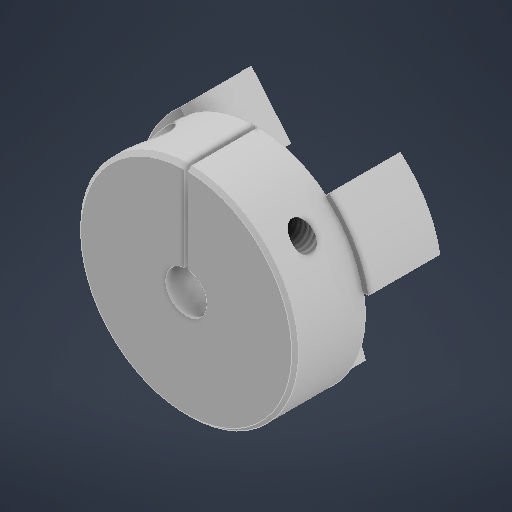
# Autodesk Inventor part: Coupling
Saved by Autodesk Inventor 2027 (Build 310192000, 192)
## iProperties
Category: PARTsolutions
Company: FESTO
Created: 2026-05-27
Part Number: Coupling
Material: Generic
Catalog Web Link: www.3dfindit.com
Description: EAMD-coupling
Vendor: FESTO
Document SubType Name: Modeling
Designer: psAdmin
Manufacturer: FESTO
Mass: 126 g
Surface Area: 117.587 cm^2
Volume: 24.6259 cm^3
Density: 1 g/cm^3
Appearance: PSOLRGB-176-176-176
PSOL_IDENT_0: {$CADENAS_DATA/23d-libs/festo/parts/e/eamd/eamd.prj},190 {VTYP=3D},{NB=558001 EAMD-32-32-11-16x20},{
PSOL_IDENT_1: LINA=558001 EAMD-32-32-11-16x20},{NN=EAMD},{DATE=05.05.2026 07:51:46},{GEOMDATE=01.09.2025 08:29:23}
PSOL_IDENT_2: ,{VERSION=},{LINEID=40},{WBVAR=},{WBNUMERIC=}  {NB=558001 EAMD-32-32-11-16x20},{LINA=558001 EAMD-32-
PSOL_IDENT_3: 32-11-16x20},{KT=DUMMY},{TNR=558001},{TYP=EAMD-32-32-11-16x20},{INFO=},{D1=11.000},{D2=16.000},{DA=0
PSOL_IDENT_4: .000},{F=0.000},{L1=0.000},{L2=0.000},{L3=0.000},{L4=0.000},{L5=0.000},{A=3.950},{VERS=3},{CNSMASSEX
PSOL_IDENT_5: ACT=0.1260},{GTIN=4052568204419},{EOLDATE=}
NB: 558001 EAMD-32-32-11-16x20
NN: EAMD
NT: coupling
NBSYN: $TNR. $TYP.
LINA: 558001 EAMD-32-32-11-16x20
CATALOG: Festo
TNR: 558001
TYP: EAMD-32-32-11-16x20
D1: 11
D2: 16
DA: 0
F: 0
L1: 0
L2: 0
L3: 0
L4: 0
L5: 0
CNSMASSEXACT: 0.126
GTIN: 4052568204419
SUPPLIER: FESTO
ARTICLENO: 558001 EAMD-32-32-11-16x20
BOMINFO: 558001 EAMD-32-32-11-16x20
CREATOR: CADENAS GmbH
Title: 558001 EAMD-32-32-11-16x20
Author: Cadenas PARTsolutions
Comments: coupling
Autodesk Inventor part; units mm, degrees
sketch "Sketch_1" plane through (0, 0, 0) normal (1, 0, 0) x (0, 1, 0)
  line L0 (0, -10.3) -> (0, 0)
  line L1 (0, 0) -> (15.5, 0)
  line L2 (15.5, 0) -> (16, -0.5)
  line L3 (16, -0.5) -> (16, -10.3)
  line L4 (16, -10.3) -> (0, -10.3)
  line L5 (0, -10.3) -> (0, 0)
  constraints: 12 end point
revolve "Revolution1" add sketch "Sketch_1" angle 360 about axis through (0, 0, -10.3) along (0, 0, -1)
sketch "Sketch_2" plane through (0, 0, -10.1) normal (0, 0, 1) x (1, 0, 0)
  line L0 (-16.7417, 2.952) -> (-7.8785, 1.3892)
  arc A0 (-5.1423, 6.1284) -> (-7.8785, 1.3892) centre (0, 0) ccw
  line L1 (-5.1423, 6.1284) -> (-10.9274, 13.0228)
  arc A1 (-10.9274, 13.0228) -> (-16.7417, 2.952) centre (0, 0) ccw
  constraints: 4 end point, 4 point on circle, 2 centre point
extrude "Extrusion1" add sketch "Sketch_2" against normal blind 10.4
sketch "Sketch_3" plane through (0, 0, -10.1) normal (0, 0, 1) x (1, 0, 0)
  arc A0 (-5.8143, -15.9748) -> (5.8143, -15.9748) centre (0, 0) ccw
  line L0 (5.8143, -15.9748) -> (2.7362, -7.5175)
  arc A1 (-2.7362, -7.5175) -> (2.7362, -7.5175) centre (0, 0) ccw
  line L1 (-2.7362, -7.5175) -> (-5.8143, -15.9748)
  constraints: 4 end point, 4 point on circle, 2 centre point
extrude "Extrusion2" add sketch "Sketch_3" against normal blind 10.4
sketch "Sketch_19" plane through (0, 0, -10.1) normal (0, 0, 1) x (1, 0, 0)
  arc A0 (7.8785, 1.3892) -> (5.1423, 6.1284) centre (0, 0) ccw
  line L0 (7.8785, 1.3892) -> (16.7417, 2.952)
  arc A1 (16.7417, 2.952) -> (10.9274, 13.0228) centre (0, 0) ccw
  line L1 (10.9274, 13.0228) -> (5.1423, 6.1284)
  constraints: 4 end point, 4 point on circle, 2 centre point
extrude "Extrusion3" add sketch "Sketch_19" against normal blind 10.4
sketch "Sketch_9" plane through (0, 0, 0) normal (1, 0, 0) x (0, 1, 0)
  line L0 (0, -28.3636) -> (0, 0)
  line L1 (0, 0) -> (3, 0)
  line L2 (3, 0) -> (3, -5.5091)
  line L3 (3, -5.5091) -> (3.8727, -5.5091)
  line L4 (3.8727, -5.5091) -> (3.8727, -11.8909)
  line L5 (3.8727, -11.8909) -> (2.4545, -11.8909)
  line L6 (2.4545, -11.8909) -> (2.4545, -13.2545)
  line L7 (2.4545, -13.2545) -> (1.1275, -13.2545)
  line L8 (1.1275, -13.2545) -> (1.1275, -28.1275)
  line L9 (1.1275, -28.1275) -> (1.3636, -28.3636)
  line L10 (1.3636, -28.3636) -> (0, -28.3636)
  line L11 (0, -28.3636) -> (0, 0)
  dimension "d36" = 3
  constraints: 24 end point
  measures "d36" distance of L1.start L1.end
revolve "Revolution3" cut sketch "Sketch_9" angle 360 about axis through (0, 0, -28.3636) along (0, 0, -1)
sketch "Sketch_12" plane through (0, 0, 0) normal (0, 0, 1) x (1, 0, 0)
  line L0 (-0.25, 16) -> (-0.25, 0)
  line L1 (-0.25, 0) -> (0.25, 0)
  line L2 (0.25, 0) -> (0.25, 16)
  line L3 (0.25, 16) -> (-0.25, 16)
  constraints: 8 end point
extrude "Extrusion10" cut sketch "Sketch_12" against normal blind 10.1
sketch "Sketch_13" plane through (0, 0, -5.1) normal (0, 0, 1) x (1, 0, 0)
  line L0 (13.5, 10.5) -> (-16.5, 10.5)
  line L1 (-16.5, 10.5) -> (-16.5, 14.1)
  line L2 (-16.5, 14.1) -> (-4.5, 14.1)
  line L3 (-4.5, 14.1) -> (-4.5, 12.5)
  line L4 (-4.5, 12.5) -> (-4.121, 12.121)
  line L5 (-4.121, 12.121) -> (13.5, 12.121)
  line L6 (13.5, 12.121) -> (13.5, 10.5)
  line L7 (13.5, 10.5) -> (-16.5, 10.5)
  constraints: 16 end point
revolve "Revolution6" cut sketch "Sketch_13" angle 360 about axis through (13.5, 10.5, -5.1) along (-1, 0, 0)
thread "Thread2" size "M4x0.7" class "6H" standard "ISO Metric profile" length 17.621
sketch "Sketch_11" plane through (0, 0, -21.8) normal (0, 0, 1) x (0, 1, 0)
  arc A0 (-1.8674, -0.5726) -> (-1.4296, -1.3309) centre (-1.5586, -0.8998) ccw
  arc A1 (-0.4378, -1.9035) -> (-1.4296, -1.3309) centre (-1.2039, -2.0852) ccw
  arc A2 (-0.4378, -1.9035) -> (0.4378, -1.9035) centre (0, -1.7997) ccw
  arc A3 (1.4296, -1.3309) -> (0.4378, -1.9035) centre (1.2039, -2.0852) ccw
  arc A4 (1.4296, -1.3309) -> (1.8674, -0.5726) centre (1.5586, -0.8998) ccw
  arc A5 (1.8674, 0.5726) -> (1.8674, -0.5726) centre (2.4078, 0) ccw
  arc A6 (1.8674, 0.5726) -> (1.4296, 1.3309) centre (1.5586, 0.8999) ccw
  arc A7 (0.4378, 1.9035) -> (1.4296, 1.3309) centre (1.2039, 2.0852) ccw
  arc A8 (0.4378, 1.9035) -> (-0.4378, 1.9035) centre (0, 1.7997) ccw
  arc A9 (-1.4296, 1.3309) -> (-0.4378, 1.9035) centre (-1.2039, 2.0852) ccw
  arc A10 (-1.4296, 1.3309) -> (-1.8674, 0.5726) centre (-1.5586, 0.8999) ccw
  arc A11 (-1.8674, -0.5726) -> (-1.8674, 0.5726) centre (-2.4078, 0) ccw
  constraints: 24 point on circle, 12 centre point
extrude "Extrusion11" cut sketch "Sketch_11" against normal blind 2.64
sketch "Sketch_15" plane through (-8.5, 10.5, -5.1) normal (-1, 0, 0) x (0, 1, 0)
  arc A0 (-1.6394, -0.5027) -> (-1.2551, -1.1684) centre (-1.3683, -0.79) ccw
  arc A1 (-0.3843, -1.6711) -> (-1.2551, -1.1684) centre (-1.0569, -1.8307) ccw
  arc A2 (-0.3843, -1.6711) -> (0.3843, -1.6711) centre (0, -1.58) ccw
  arc A3 (1.2551, -1.1684) -> (0.3843, -1.6711) centre (1.0569, -1.8307) ccw
  arc A4 (1.2551, -1.1684) -> (1.6394, -0.5027) centre (1.3683, -0.79) ccw
  arc A5 (1.6394, 0.5027) -> (1.6394, -0.5027) centre (2.1139, 0) ccw
  arc A6 (1.6394, 0.5027) -> (1.2551, 1.1684) centre (1.3683, 0.79) ccw
  arc A7 (0.3843, 1.6711) -> (1.2551, 1.1684) centre (1.0569, 1.8307) ccw
  arc A8 (0.3843, 1.6711) -> (-0.3843, 1.6711) centre (0, 1.58) ccw
  arc A9 (-1.2551, 1.1684) -> (-0.3843, 1.6711) centre (-1.0569, 1.8307) ccw
  arc A10 (-1.2551, 1.1684) -> (-1.6394, 0.5027) centre (-1.3683, 0.79) ccw
  arc A11 (-1.6394, -0.5027) -> (-1.6394, 0.5027) centre (-2.1139, 0) ccw
  constraints: 24 point on circle, 12 centre point
extrude "Extrusion12" cut sketch "Sketch_15" against normal blind 2.34
ref_plane "KUPPLUNG_XY" through (0, 0, 0) normal (0, 0, 1) x (1, 0, 0)
ref_plane "KUPPLUNG_YZ" through (0, 0, 0) normal (1, 0, 0) x (0, 1, 0)
ref_plane "KUPPLUNG_ZX" through (0, 0, 0) normal (0, 1, 0) x (0, 0, 1)
body "Solid1"
